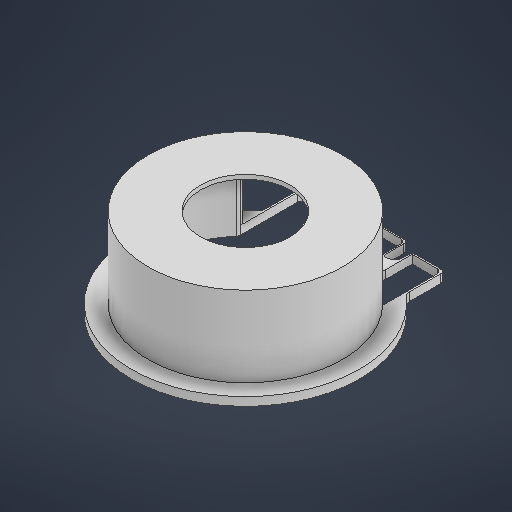
# Autodesk Inventor part: Cylinder  Segment - 01
Saved by Autodesk Inventor 2025 (Build 290162000, 162)
## iProperties
Created: 2024-04-11
Part Number: Cylinder  Segment - 01
Material: Generic
Document SubType Name: Modeling
Designer: Thienan Hoang
Density: 1 g/cm^3
Appearance: Default
Author: Thienan Hoang
Autodesk Inventor part; units mm, degrees
ref_plane "YZ Plane" through (0, 0, 0) normal (1, 0, 0) x (0, 1, 0)
ref_plane "XZ Plane" through (0, 0, 0) normal (0, 1, 0) x (-1, 0, 0)
ref_plane "XY Plane" through (0, 0, 0) normal (0, 0, 1) x (1, 0, 0)
sketch "Sketch1" plane through (0, 0, 0) normal (0, 1, 0) x (-1, 0, 0)
  circle A0 centre (0, 0) radius 135
  circle A1 centre (0, 0) radius 115
  circle A2 centre (0, 0) radius 112.0375
  circle A3 centre (0, 0) radius 9.5
  dimension "Absolute_Diameter" = 270
  dimension "Diameter_No_Outer_Lip" = 230
  dimension "Inner_Cylinder_Diameter" = 224.075
  dimension "Lip_Diameter" = 19
  constraints: 4 centre point, 4 coincident
  measures "Absolute_Diameter" diameter of A0
  measures "Diameter_No_Outer_Lip" diameter of A1
  measures "Inner_Cylinder_Diameter" diameter of A2
  measures "Lip_Diameter" diameter of A3
extrude "Extrusion1" add sketch "Sketch1" along normal blind 10 contours A0
extrude "Extrusion2" add sketch "Sketch1" along normal blind 105 contours A1
sketch "Sketch2" plane through (0, 105, 0) normal (0, 1, 0) x (1, 0, 0)
  circle A0 centre (0, 0) radius 115
  circle A1 centre (0, 0) radius 53.125
  dimension "Lip_Diameter_Out" = 230
  dimension "Inner_Lip_Diameter" = 106.25
  constraints: 2 centre point, 1 coincident
  measures "Lip_Diameter_Out" diameter of A0
  measures "Inner_Lip_Diameter" diameter of A1
extrude "Extrusion7" add sketch "Sketch2" against normal blind 5
sketch "Sketch24" plane through (0, 0, 0) normal (0, -1, 0) x (1, 0, 0)
  circle A0 centre (0, 0) radius 112.0375
  arc A1 (-85.157, -104.7535) -> (32.5, -131.0296) centre (0, 0) ccw
  circle A2 centre (0, 0) radius 133
  line L0 (-32.5, -70.125) -> (32.5, -70.125)
  line L1 (32.5, -70.125) -> (32.5, -160.125)
  line L2 (32.5, -160.125) -> (-32.5, -160.125)
  line L3 (-32.5, -160.125) -> (-32.5, -70.125)
  line L4 (-31, -158.625) -> (31, -158.625)
  line L5 (31, -158.625) -> (31, -71.625)
  line L6 (31, -71.625) -> (-31, -71.625)
  line L7 (-31, -71.625) -> (-31, -158.625)
  line L8 (-85.157, -65.125) -> (-46.3, -65.125)
  line L9 (-46.3, -65.125) -> (-46.3, -151.2985)
  line L10 (-46.3, -151.2985) -> (-85.157, -151.2985)
  line L11 (-85.157, -151.2985) -> (-85.157, -65.125)
  arc A3 (32.5, -131.0296) -> (-85.157, -104.7535) centre (0, 0) ccw
  line L12 (0, -71.625) -> (0, -158.625)
  line L13 (-83.157, -149.2985) -> (-48.3, -149.2985)
  line L14 (-48.3, -149.2985) -> (-48.3, -67.125)
  line L15 (-48.3, -67.125) -> (-83.157, -67.125)
  line L16 (-83.157, -67.125) -> (-83.157, -149.2985)
  line L17 (85.157, -65.125) -> (46.3, -65.125)
  line L18 (46.3, -65.125) -> (46.3, -151.2985)
  line L19 (46.3, -151.2985) -> (85.157, -151.2985)
  line L20 (85.157, -151.2985) -> (85.157, -65.125)
  line L21 (83.157, -149.2985) -> (48.3, -149.2985)
  line L22 (48.3, -149.2985) -> (48.3, -67.125)
  line L23 (48.3, -67.125) -> (83.157, -67.125)
  line L24 (83.157, -67.125) -> (83.157, -149.2985)
  circle A4 centre (0, 0) radius 120
  point P0 (0, -135)
  point P1 (48.3, -126.0639)
  point P2 (83.157, -106.3481)
  point P3 (-31, -131.3925)
  point P4 (31, -131.3925)
  point P5 (-83.157, -106.3481)
  point P6 (-48.3, -126.0639)
  point P7 (46.3, -126.8121)
  point P8 (85.157, -104.7535)
  point P9 (-32.5, -131.0296)
  point P10 (-46.3, -126.8121)
  point P11 (48.3, -109.8504)
  point P12 (48.3, -101.0916)
  point P13 (31, -107.6634)
  point P14 (31, -115.9267)
  point P15 (-48.3, -109.8504)
  point P16 (-31, -115.9267)
  point P17 (-31, -107.6634)
  point P18 (-48.3, -101.0916)
  dimension "d234" = 2
  dimension "d235" = 65
  dimension "d237" = 1.5
  dimension "d238" = 65.125
  dimension "d240" = 20.9625
  dimension "d241" = 270
  dimension "d242" = 70.125
  dimension "d243" = 13.8
  dimension "d244" = 38.857
  dimension "d247" = 2
  dimension "d248" = 90
  dimension "d253" = 240
  constraints: 50 end point, 8 parallel, 8 symmetric about line, 5 centre point, 5 point on circle, 4 perpendicular, 3 coincident, 2 horizontal, 2 midpoint, 2 point on line, 6 other
  measures "d234" radial gap between concentric circles of A1 A2
  measures "d235" distance of L1.end L2.end
  measures "d237" distance between parallel lines of L2 L4
  measures "d238" distance from line of point (0, 0) L8
  measures "d240" radial gap between concentric circles of A2 A0
  measures "d241" diameter of A1
  measures "d242" distance from line of A0.centre L0
  measures "d243" distance between parallel lines of L3 L9
  measures "d244" distance of L9.end L10.end
  measures "d247" distance between parallel lines of L10 L13
  measures "d248" distance of L2.end L0.start
  measures "d253" diameter of A4
extrude "Extrusion30" cut sketch "Sketch24" against normal blind 93 contours L16 L15 L14 A0 | A0 L14 A4 L16 | L24 A4 L22 A0 | A0 L22 L23 L24 | A4 L14 A2 L16 | L24 A2 L22 A4 | A2 L14 A1 L16 | L24 A3 L22 A2 | L7 L6 L12 A0 | A0 L12 A4 L7 | L5 A4 L12 A0 | A0 L12 L6 L5 | A4 L12 A2 L7 | L5 A2 L12 A4 | A2 L12 A1 L7 | L5 A1 L12 A2
extrude "Extrusion31" add sketch "Sketch24" against normal up to surface (10 mm away) contours A1 L16 L13 L14 L9 L10 L11 | L20 L19 L18 A3 L22 L21 L24 | A1 L7 L4 L5 L1 L2 L3
extrude "Extrusion32" cut sketch "Sketch24" against normal up to surface (93 mm away) contours A0 L9 A4 L14 | L22 A4 L18 A0 | A0 L3 A4 L9 | L18 A4 L1 A0 | A0 L7 A4 L3 | L1 A4 L5 A0
fillet "Fillet14" radius 10 2 edges at (85.157, 5, -104.7535) (-85.157, 5, -104.7535)
fillet "Fillet15" radius 10 2 edges at (-46.3, 5, -126.8121) (46.3, 5, -126.8121)
fillet "Fillet16" radius 2 2 edges at (32.5, 5, -131.0296) (-32.5, 5, -131.0296)
fillet "Fillet17" radius 5 6 edges at (-85.157, 5, -151.2985) (-46.3, 5, -151.2985) (-32.5, 5, -160.125) (32.5, 5, -160.125) (46.3, 5, -151.2985) (85.157, 5, -151.2985)
fillet "Fillet18" radius 5 11 edges at (31, 5, -158.625) (83.157, 5, -149.2985) (-31, 5, -158.625) (-48.3, 5, -149.2985) (-83.157, 5, -149.2985) (31, 5, -115.9267) (48.3, 5, -109.8504) (-31, 5, -115.9267) (-48.3, 5, -109.8504) (83.157, 46.5, -75.0821) (-83.157, 46.5, -75.0821)
body "Solid1"
